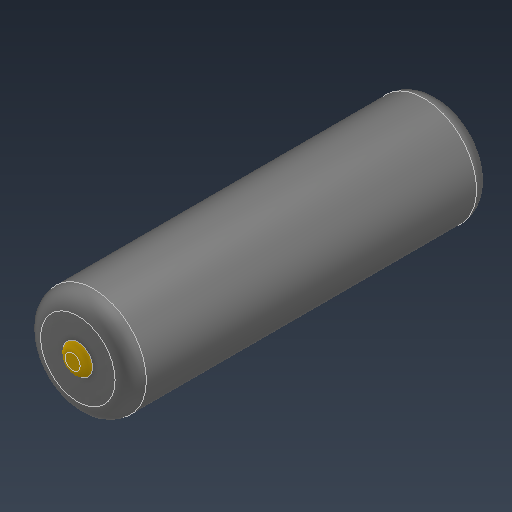
# Autodesk Inventor part: Battery
Saved by Autodesk Inventor 2025.1 (Build 291241000, 241)
## iProperties
Created: 2023-04-25
Part Number: Battery
Material: Generic
Vendor: The Saber Armory
Document SubType Name: Modeling
Designer: Michael
Density: 1 g/cm^3
Appearance: Default
Author: Michael
Sending System: SolidWorks 2022
Last Author: foams
Last Saved: 2023-04-27
Part Name: KeepPower 21700 Rechargeable
Autodesk Inventor part; units mm, degrees
ref_plane "YZ Plane" through (0, 0, 0) normal (1, 0, 0) x (0, 1, 0)
ref_plane "XZ Plane" through (0, 0, 0) normal (0, 1, 0) x (-1, 0, 0)
ref_plane "XY Plane" through (0, 0, 0) normal (0, 0, 1) x (1, 0, 0)
sketch "Sketch1" plane through (0, 0, 0) normal (0, 0, 1) x (1, 0, 0)
  circle A0 centre (0, 0) radius 10.75 projected
  circle A1 centre (0, 0) radius 10.75 projected
  circle A2 centre (0, 0) radius 3 projected
  circle A3 centre (0, 0) radius 7.5 projected
extrude "Extrusion1" add sketch "Sketch1" along normal blind 73.4568 contours A0 | A2 | A3
extrude "Extrusion2" cut sketch "Sketch1" along normal blind 0.0508 contours A2 | A3
extrude "Extrusion3" add sketch "Sketch1" along normal blind 1.0414 from surface at 73.4568 contours A2
fillet "Fillet1" radius 3.175 2 edges at (-10.75, 0, 73.4568) (-10.75, 0, 0)
fillet "Fillet2" radius 1.5875 1 edges at (-3, 0, 74.4982)
body "Solid1"
